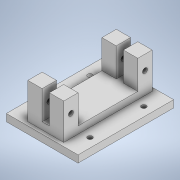
# Autodesk Inventor part: camera_plate2
Saved by Autodesk Inventor 2020 (Build 240168000, 168)
## iProperties
Created: 2020-02-09
Part Number: camera_plate2
Material: Generic
Document SubType Name: Modeling
Designer: mdjb501
Density: 1 g/cm^3
Appearance: Default
Author: mdjb501
Autodesk Inventor part; units mm, degrees
ref_plane "YZ Plane" through (0, 0, 0) normal (1, 0, 0) x (0, 1, 0)
ref_plane "XZ Plane" through (0, 0, 0) normal (0, 1, 0) x (-1, 0, 0)
ref_plane "XY Plane" through (0, 0, 0) normal (0, 0, 1) x (1, 0, 0)
sketch "Sketch1" plane through (0, 0, 0) normal (0, 1, 0) x (-1, 0, 0)
  circle A0 centre (11.25, 11.25) radius 1
  circle A1 centre (11.25, -11.25) radius 1
  circle A2 centre (-11.25, 11.25) radius 1
  circle A3 centre (-11.25, -11.25) radius 1
  line L0 (-7.5, -18.5) -> (7.5, -18.5)
  line L1 (7.5, -18.5) -> (7.5, 18.5)
  line L2 (7.5, 18.5) -> (-7.5, 18.5)
  line L3 (-7.5, 18.5) -> (-7.5, -18.5)
  line L4 (-15, -20) -> (15, -20)
  line L5 (15, -20) -> (15, 20)
  line L6 (15, 20) -> (-15, 20)
  line L7 (-15, 20) -> (-15, -20)
  line L8 (7.5, -18.5) -> (1.5, -18.5)
  line L9 (1.5, -18.5) -> (1.5, -12.5)
  line L10 (1.5, -12.5) -> (7.5, -12.5)
  line L11 (7.5, -12.5) -> (7.5, -18.5)
  line L12 (-7.5, -18.5) -> (-1.5, -18.5)
  line L13 (-1.5, -18.5) -> (-1.5, -12.5)
  line L14 (-1.5, -12.5) -> (-7.5, -12.5)
  line L15 (-7.5, -12.5) -> (-7.5, -18.5)
  line L16 (-7.5, 18.5) -> (-1.5, 18.5)
  line L17 (-1.5, 18.5) -> (-1.5, 12.5)
  line L18 (-1.5, 12.5) -> (-7.5, 12.5)
  line L19 (-7.5, 12.5) -> (-7.5, 18.5)
  line L20 (7.5, 18.5) -> (1.5, 18.5)
  line L21 (1.5, 18.5) -> (1.5, 12.5)
  line L22 (1.5, 12.5) -> (7.5, 12.5)
  line L23 (7.5, 12.5) -> (7.5, 18.5)
  point P0 (0, 0)
  constraints: 48 end point, 12 parallel, 6 horizontal, 6 perpendicular, 4 centre point
extrude "Extrusion7" add sketch "Sketch1" along normal blind 18 contours L3 L14 L13 L0 | L9 L10 L1 L0 | L3 L2 L17 L18 | L22 L21 L2 L1
extrude "Extrusion8" add sketch "Sketch1" along normal blind 6 contours L13 L14 L3 L18 L17 L2 L21 L22 L1 L10 L9 L0
extrude "Extrusion9" add sketch "Sketch1" along normal blind 3
sketch "Sketch4" plane through (-7.5, 18, 12.5) normal (-1, 0, 0) x (0, 0, 1)
  line L0 (-25, -12) -> (-31, -12) projected
  line L1 (-28, -12) -> (-28, -6)
  line L2 (6, -12) -> (0, -12) projected
  line L3 (3, -12) -> (3, -6)
  circle A0 centre (-28, -6) radius 1.05
  circle A1 centre (3, -6) radius 1.05
  point P0 (-12.5, -18)
  dimension "d65" = 6
  dimension "d66" = 6
  dimension "d67" = 2.1
  dimension "d68" = 2.1
  constraints: 4 end point, 2 centre point, 2 coincident, 2 midpoint, 2 vertical
  measures "d65" distance of L1.start L1.end
  measures "d66" distance of L3.start L3.end
  measures "d67" diameter of A0
  measures "d68" diameter of A1
extrude "Extrusion10" cut sketch "Sketch4" against normal blind 18
body "Solid2"
